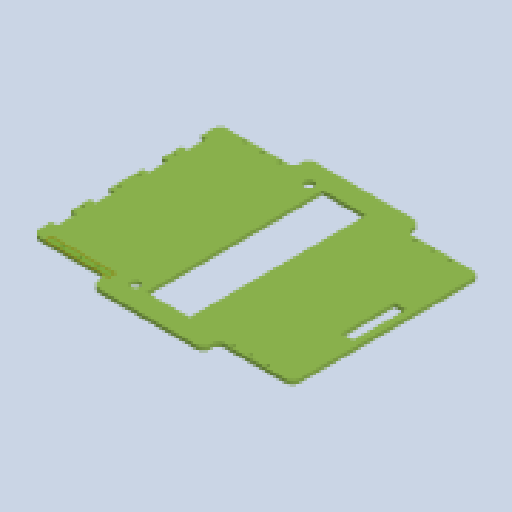
# Autodesk Inventor part: верхняя пластина
Saved by Autodesk Inventor 2024.2 (Build 282272000, 272)
## iProperties
Created: 2025-11-23
Part Number: верхняя пластина
Material: Типовые
Document SubType Name: Modeling
Designer: katya_notebook
Density: 1 g/cm^3
Appearance: Оливково-зеленый
Mass: 177.745 g
Surface Area: 959.322 cm^2
Volume: 177.745 cm^3
Author: katya_notebook
Autodesk Inventor part; units mm, degrees
ref_plane "YZ Plane" through (0, 0, 0) normal (1, 0, 0) x (0, 1, 0)
ref_plane "XZ Plane" through (0, 0, 0) normal (0, 1, 0) x (-1, 0, 0)
ref_plane "XY Plane" through (0, 0, 0) normal (0, 0, 1) x (1, 0, 0)
ref_plane "РабПлоскость1" through (-487.5503, -280.3956, -187.6025) normal (0, -1, 0) x (1, 0, 0)
sketch "Эскиз1" plane through (-487.5503, -280.3956, -187.6025) normal (0, -1, 0) x (1, 0, 0)
  line L0 (-76.4763, 6.5) -> (193.5237, 6.5)
  line L1 (193.5237, 6.5) -> (193.5237, -188.5)
  line L2 (193.5237, -188.5) -> (-76.4763, -188.5)
  line L3 (-76.4763, -188.5) -> (-76.4763, 6.5)
  line L4 (-76.4763, -13.5) -> (-76.4763, -1.5) projected
  circle A0 centre (-12, 3.25) radius 1.75
  circle A1 centre (-48, 3.25) radius 1.75
  circle A2 centre (-30, 3.25) radius 1.75
  line L5 (-76.4763, -91) -> (193.5237, -91)
  circle A3 centre (-12, -185.25) radius 1.75
  circle A4 centre (-48, -185.25) radius 1.75
  circle A5 centre (-30, -185.25) radius 1.75
  point P0 (487.5503, 187.6025)
  point P1 (-60, 3.25)
  dimension "d0" = 195
  dimension "d1" = 270
  dimension "d2" = 0
  dimension "d5" = 3.5
  dimension "d6" = 3.5
  dimension "d8" = 12
  dimension "d9" = 3.25
  dimension "d10" = 3.25
  dimension "d11" = 3.5
  dimension "d12" = 3.25
  dimension "d13" = 18
  dimension "d14" = 97.5
  constraints: 10 end point, 6 centre point, 3 symmetric about line, 2 parallel, 2 perpendicular, 1 horizontal, 1 midpoint, 1 point on line, 3 other
  measures "d0" distance of L0.end L1.end
  measures "d1" distance of L1.end L2.end
  measures "d2" distance between parallel lines of L4 L3
  measures "d5" diameter of A1
  measures "d6" diameter of A0
  measures "d8" distance of A1.centre point (-60, 3.25)
  measures "d9" distance from line of L0 A0.centre
  measures "d10" distance from line of L0 A1.centre
  measures "d11" diameter of A2
  measures "d12" distance from line of L0 A2.centre
  measures "d13" distance of A1.centre A2.centre
  measures "d14" distance between parallel lines of L5 L0
extrude "Выдавливание1" add sketch "Эскиз1" along normal blind 4 contours L0 L1 L5 L3 | L1 L2 L3 L5 | A0 | A1 | A2 | A3 | A4 | A5
sketch "Эскиз2" plane through (-487.5503, -284.3956, -187.6025) normal (0, -1, 0) x (1, 0, 0)
  circle A0 centre (-48, -185.25) radius 1.75 projected
  circle A1 centre (-30, -185.25) radius 1.75 projected
  circle A2 centre (-12, -185.25) radius 1.75 projected
  line L0 (0, -182) -> (-60, -182) projected
  line L1 (-60, -182) -> (-60, -188.5) projected
  line L2 (0, -188.5) -> (-60, -188.5) projected
  line L3 (0, -182) -> (0, -188.5) projected
  circle A3 centre (-48, 3.25) radius 1.75 projected
  circle A4 centre (-30, 3.25) radius 1.75 projected
  circle A5 centre (-12, 3.25) radius 1.75 projected
  line L4 (0, 0) -> (-60, 0) projected
  line L5 (0, 0) -> (0, 6.5) projected
  line L6 (0, 6.5) -> (-60, 6.5) projected
  line L7 (-60, 0) -> (-60, 6.5) projected
  circle A6 centre (165.0475, 3.25) radius 1.75 projected
  circle A7 centre (129.0475, 3.25) radius 1.75 projected
  circle A8 centre (147.0475, 3.25) radius 1.75 projected
  line L8 (116.803, 6.5) -> (116.803, 0) projected
  line L9 (116.803, 0) -> (176.803, 0) projected
  line L10 (176.803, 0) -> (176.803, 6.5) projected
  line L11 (176.803, 6.5) -> (116.803, 6.5) projected
  circle A9 centre (165.0475, -185.25) radius 1.75 projected
  circle A10 centre (129.0475, -185.25) radius 1.75 projected
  circle A11 centre (147.0475, -185.25) radius 1.75 projected
  line L12 (116.803, -188.5) -> (116.803, -182) projected
  line L13 (176.803, -188.5) -> (116.803, -188.5) projected
  line L14 (176.803, -182) -> (176.803, -188.5) projected
  line L15 (116.803, -182) -> (176.803, -182) projected
  line L16 (81.0237, 0.5) -> (81.0237, -182.5) projected
  line L17 (36.0237, 0.5) -> (81.0237, 0.5) projected
  line L18 (36.0237, -182.5) -> (36.0237, 0.5) projected
  line L19 (36.0237, -182.5) -> (81.0237, -182.5) projected
  point P0 (487.5503, 187.6025)
extrude "Выдавливание2" cut sketch "Эскиз2" against normal blind 10 contours A0 | A1 | A2 | A3 | A4 | A5 | A6 | A7 | A8 | A9 | A10 | A11
sketch "Эскиз3" plane through (-487.5503, -284.3956, -187.6025) normal (0, -1, 0) x (1, 0, 0)
  circle A0 centre (23.5237, -1) radius 5 projected
  circle A1 centre (23.5237, -181) radius 5 projected
  line L0 (36.0237, -182.5) -> (36.0237, 0.5) projected
  line L1 (81.0237, 0.5) -> (81.0237, -182.5) projected
  line L2 (36.0237, 0.5) -> (81.0237, 0.5) projected
  line L3 (81.0237, -182.5) -> (36.0237, -182.5) projected
  point P0 (487.5503, 187.6025)
extrude "Выдавливание3" cut sketch "Эскиз3" against normal blind 10
sketch "Эскиз4" plane through (-487.5503, -284.3956, -187.6025) normal (0, -1, 0) x (1, 0, 0)
  arc A0 (116.803, 10.7701) -> (120.803, 6.5) centre (124.2371, 13.7254) ccw projected
  line L0 (116.803, 10.7701) -> (0.2701, 10.7701) projected
  arc A1 (-4, 6.5) -> (0.2701, 10.7701) centre (-7.1034, 13.8735) ccw projected
  arc A2 (0, -192.5) -> (-4, -188.5) centre (-7.2915, -195.7915) ccw projected
  line L1 (0, -192.5) -> (116.803, -192.5) projected
  arc A3 (120.803, -188.5) -> (116.803, -192.5) centre (124.0945, -195.7915) ccw projected
  line L2 (120.803, -188.5) -> (-4, -188.5)
  line L3 (-4, 6.5) -> (120.803, 6.5)
  point P0 (487.5503, 187.6025)
  constraints: 4 end point, 1 horizontal, 1 parallel
extrude "Выдавливание4" add sketch "Эскиз4" against normal blind 4
sketch "Эскиз5" plane through (-487.5503, -284.3956, -187.6025) normal (0, -1, 0) x (1, 0, 0)
  line L0 (174.5237, -118.4235) -> (174.5237, -63.4235) projected
  line L1 (186.5237, -118.4235) -> (174.5237, -118.4235) projected
  line L2 (186.5237, -63.4235) -> (186.5237, -118.4235) projected
  line L3 (174.5237, -63.4235) -> (186.5237, -63.4235) projected
  point P0 (487.5503, 187.6025)
extrude "Выдавливание5" cut sketch "Эскиз5" against normal blind 10
ref_plane "РабПлоскость2" through (-558.0266, -285.3956, -376.1025) normal (1, 0, 0) x (0, 1, 0)
sketch "Эскиз7" plane through (-564.0266, -280.3956, -376.1025) normal (-1, 0, 0) x (0, 0, 1)
  line L0 (175, -5) -> (175, 0) projected
  line L1 (155, 0) -> (155, -5) projected
  line L2 (155, -5) -> (175, -5) projected
  line L3 (195, 0) -> (0, 0) projected
  line L4 (115, -5) -> (135, -5) projected
  line L5 (135, -5) -> (135, 0) projected
  line L6 (115, 0) -> (115, -5) projected
  line L7 (80, -5) -> (80, 0) projected
  line L8 (60, -5) -> (80, -5) projected
  line L9 (60, 0) -> (60, -5) projected
  line L10 (40, -5) -> (40, 0) projected
  line L11 (20, -5) -> (40, -5) projected
  line L12 (20, 0) -> (20, -5) projected
  line L13 (90.375, 55.705) -> (90.375, 55.205) projected
  line L14 (90.375, 55.205) -> (88.875, 55.205) projected
  line L15 (85.375, 55.205) -> (83.875, 55.205) projected
  line L16 (83.875, 55.205) -> (83.875, 55.705) projected
  line L17 (80, 59.705) -> (80, 60.705) projected
  line L18 (80, 60.705) -> (60, 60.705) projected
  line L19 (60, 60.705) -> (60, 59.705) projected
  line L20 (51.75, 55.205) -> (51.75, 47.705) projected
  line L21 (53.25, 55.705) -> (53.25, 55.205) projected
  line L22 (53.25, 55.205) -> (51.75, 55.205) projected
  line L23 (51.75, 47.705) -> (48.25, 47.705) projected
  line L24 (48.25, 47.705) -> (48.25, 55.205) projected
  line L25 (48.25, 55.205) -> (46.75, 55.205) projected
  line L26 (46.75, 55.205) -> (46.75, 55.705) projected
  line L27 (40, 59.705) -> (40, 60.705) projected
  line L28 (40, 60.705) -> (20, 60.705) projected
  line L29 (20, 60.705) -> (20, 59.705) projected
  line L30 (0, 59.705) -> (0, 0) projected
  line L31 (20, 0) -> (0, 0) projected
  line L32 (20, 0) -> (20, -5) projected
  line L33 (20, -5) -> (40, -5) projected
  line L34 (40, -5) -> (40, 0) projected
  line L35 (48.25, 0) -> (40, 0) projected
  line L36 (48.25, 0) -> (48.25, 1.5) projected
  line L37 (48.25, 1.5) -> (46.75, 1.5) projected
  line L38 (46.75, 1.5) -> (46.75, 4.5) projected
  line L39 (46.75, 4.5) -> (48.25, 4.5) projected
  line L40 (48.25, 4.5) -> (48.25, 12) projected
  line L41 (48.25, 12) -> (51.75, 12) projected
  line L42 (51.75, 12) -> (51.75, 4.5) projected
  line L43 (51.75, 4.5) -> (53.25, 4.5) projected
  line L44 (53.25, 4.5) -> (53.25, 1.5) projected
  line L45 (53.25, 1.5) -> (51.75, 1.5) projected
  line L46 (51.75, 1.5) -> (51.75, 0) projected
  line L47 (60, 0) -> (51.75, 0) projected
  line L48 (60, 0) -> (60, -5) projected
  line L49 (60, -5) -> (80, -5) projected
  line L50 (80, -5) -> (80, 0) projected
  line L51 (85.375, 0) -> (80, 0) projected
  line L52 (85.375, 0) -> (85.375, 1.5) projected
  line L53 (85.375, 1.5) -> (83.875, 1.5) projected
  line L54 (83.875, 1.5) -> (83.875, 4.5) projected
  line L55 (83.875, 4.5) -> (85.375, 4.5) projected
  line L56 (88.875, 1.5) -> (88.875, 0) projected
  line L57 (88.875, 4.5) -> (90.375, 4.5) projected
  line L58 (90.375, 4.5) -> (90.375, 1.5) projected
  line L59 (90.375, 1.5) -> (88.875, 1.5) projected
  line L60 (106.125, 0) -> (88.875, 0) projected
  line L61 (115, 0) -> (109.625, 0) projected
  line L62 (106.125, 0) -> (106.125, 1.5) projected
  line L63 (106.125, 1.5) -> (104.625, 1.5) projected
  line L64 (104.625, 1.5) -> (104.625, 4.5) projected
  line L65 (104.625, 4.5) -> (106.125, 4.5) projected
  line L66 (109.625, 1.5) -> (109.625, 0) projected
  line L67 (109.625, 4.5) -> (111.125, 4.5) projected
  line L68 (111.125, 4.5) -> (111.125, 1.5) projected
  line L69 (111.125, 1.5) -> (109.625, 1.5) projected
  line L70 (115, 0) -> (115, -5) projected
  line L71 (115, -5) -> (135, -5) projected
  line L72 (135, -5) -> (135, 0) projected
  line L73 (143.25, 0) -> (135, 0) projected
  line L74 (143.25, 0) -> (143.25, 1.5) projected
  line L75 (143.25, 1.5) -> (141.75, 1.5) projected
  line L76 (141.75, 1.5) -> (141.75, 4.5) projected
  line L77 (141.75, 4.5) -> (143.25, 4.5) projected
  line L78 (143.25, 4.5) -> (143.25, 12) projected
  line L79 (143.25, 12) -> (146.75, 12) projected
  line L80 (146.75, 12) -> (146.75, 4.5) projected
  line L81 (146.75, 4.5) -> (148.25, 4.5) projected
  line L82 (148.25, 4.5) -> (148.25, 1.5) projected
  line L83 (148.25, 1.5) -> (146.75, 1.5) projected
  line L84 (146.75, 1.5) -> (146.75, 0) projected
  line L85 (155, 0) -> (146.75, 0) projected
  line L86 (155, 0) -> (155, -5) projected
  line L87 (155, -5) -> (175, -5) projected
  line L88 (175, -5) -> (175, 0) projected
  line L89 (195, 0) -> (175, 0) projected
  line L90 (195, 59.705) -> (195, 0) projected
  line L91 (175, 59.705) -> (175, 60.705) projected
  line L92 (175, 60.705) -> (155, 60.705) projected
  line L93 (155, 60.705) -> (155, 59.705) projected
  line L94 (146.75, 55.205) -> (146.75, 47.705) projected
  line L95 (148.25, 55.705) -> (148.25, 55.205) projected
  line L96 (148.25, 55.205) -> (146.75, 55.205) projected
  line L97 (146.75, 47.705) -> (143.25, 47.705) projected
  line L98 (143.25, 47.705) -> (143.25, 55.205) projected
  line L99 (143.25, 55.205) -> (141.75, 55.205) projected
  line L100 (141.75, 55.205) -> (141.75, 55.705) projected
  line L101 (135, 59.705) -> (135, 60.705) projected
  line L102 (135, 60.705) -> (115, 60.705) projected
  line L103 (115, 60.705) -> (115, 59.705) projected
  line L104 (111.125, 55.705) -> (111.125, 55.205) projected
  line L105 (111.125, 55.205) -> (109.625, 55.205) projected
  line L106 (106.125, 55.205) -> (104.625, 55.205) projected
  line L107 (104.625, 55.205) -> (104.625, 55.705) projected
  line L108 (175, 55.705) -> (187, 55.705) projected
  line L109 (115, 55.705) -> (111.125, 55.705) projected
  line L110 (104.625, 55.705) -> (90.375, 55.705) projected
  line L111 (83.875, 55.705) -> (80, 55.705) projected
  line L112 (80, 55.705) -> (80, 59.705) projected
  line L113 (60, 59.705) -> (60, 55.705) projected
  line L114 (60, 55.705) -> (53.25, 55.705) projected
  line L115 (46.75, 55.705) -> (40, 55.705) projected
  line L116 (40, 55.705) -> (40, 59.705) projected
  line L117 (155, 59.705) -> (155, 55.705) projected
  line L118 (155, 55.705) -> (148.25, 55.705) projected
  line L119 (141.75, 55.705) -> (135, 55.705) projected
  line L120 (135, 55.705) -> (135, 59.705) projected
  line L121 (115, 59.705) -> (115, 55.705) projected
  line L122 (109.625, 55.205) -> (109.625, 47.705) projected
  line L123 (109.625, 47.705) -> (106.125, 47.705) projected
  line L124 (106.125, 47.705) -> (106.125, 55.205) projected
  line L125 (88.875, 55.205) -> (88.875, 47.705) projected
  line L126 (88.875, 47.705) -> (85.375, 47.705) projected
  line L127 (85.375, 47.705) -> (85.375, 53.705) projected
  line L128 (85.375, 6) -> (85.375, 12) projected
  line L129 (85.375, 12) -> (88.875, 12) projected
  line L130 (106.125, 4.5) -> (106.125, 12) projected
  line L131 (106.125, 12) -> (109.625, 12) projected
  line L132 (109.625, 12) -> (109.625, 4.5) projected
  line L133 (85.375, 6) -> (85.375, 6) projected
  line L134 (88.875, 12) -> (88.875, 4.5) projected
  line L135 (85.375, 53.705) -> (85.375, 53.705) projected
  line L136 (0, 59.705) -> (20, 59.705) projected
  line L137 (85.375, 4.5) -> (85.375, 6) projected
  line L138 (175, 59.705) -> (195, 59.705) projected
  line L139 (85.375, 53.705) -> (85.375, 55.205) projected
  point P0 (376.1025, 280.3956)
  point P1 (88.875, 49.205)
  point P2 (85.375, 49.205)
  point P3 (85.375, 9.5)
  point P4 (106.125, 9.5)
  point P5 (109.625, 9.5)
  point P6 (109.625, 6.5)
  point P7 (109.625, 49.205)
  point P8 (106.125, 49.205)
  point P9 (155, 55.705)
  point P10 (175, 55.705)
  point P11 (115, 55.705)
  point P12 (135, 55.705)
  point P13 (60, 55.705)
  point P14 (80, 55.705)
  point P15 (20, 55.705)
  point P16 (40, 55.705)
  point P17 (20, 0)
  point P18 (40, 0)
  point P19 (60, 0)
  point P20 (80, 0)
  point P21 (135, 0)
  point P22 (46.75, 47.1901)
  dimension "d0" = 195
  dimension "d1" = 270
  dimension "d2" = 0
  dimension "d5" = 3.5
  dimension "d6" = 3.5
  dimension "d8" = 12
  dimension "d9" = 3.25
  dimension "d10" = 3.25
  dimension "d11" = 3.5
  dimension "d12" = 3.25
  dimension "d13" = 18
  dimension "d14" = 97.5
extrude "Выдавливание7" cut sketch "Эскиз7" against normal up to surface (6 mm away) contours L2 L1 L3 L0 | L5 L4 L6 L3 | L7 L8 L9 L3 | L10 L11 L12 L3
sketch "Эскиз8" plane through (-487.5503, -284.3956, -187.6025) normal (0, -1, 0) x (1, 0, 0)
  line L0 (-70.4763, -45.25) -> (-76.4763, -45.25) projected
  line L1 (-76.4763, -40.25) -> (-70.4763, -40.25) projected
  line L2 (-76.4763, -45.25) -> (-76.4763, -41.75) projected
  line L3 (-76.4763, -45.25) -> (-70.4763, -45.25) projected
  line L4 (-70.4763, -41.75) -> (-70.4763, -45.25) projected
  line L5 (-76.4763, -41.75) -> (-70.4763, -41.75) projected
  line L6 (-76.4763, -103.125) -> (-76.4763, -103.125) projected
  line L7 (-76.4763, -103.125) -> (-70.4763, -103.125) projected
  line L8 (-70.4763, -103.125) -> (-70.4763, -103.125) projected
  line L9 (-76.4763, -140.25) -> (-76.4763, -136.75) projected
  line L10 (-76.4763, -140.25) -> (-70.4763, -140.25) projected
  line L11 (-70.4763, -136.75) -> (-70.4763, -140.25) projected
  line L12 (-76.4763, -136.75) -> (-70.4763, -136.75) projected
  circle A0 centre (-73.4763, -43.5) radius 1.75
  circle A1 centre (-73.4763, -80.625) radius 1.75
  circle A2 centre (-73.4763, -101.375) radius 1.75
  circle A3 centre (-73.4763, -138.5) radius 1.75
  line L13 (-76.4763, -103.125) -> (-70.4763, -103.125) projected
  point P0 (487.5503, 187.6025)
  constraints: 4 centre point
extrude "Выдавливание8" cut sketch "Эскиз8" against normal blind 10 contours A0 | A3 | A1 | A2
sketch "Эскиз9" plane through (-487.5503, -284.3956, -187.6025) normal (0, -1, 0) x (1, 0, 0)
  line L0 (0, -192.5) -> (116.803, -192.5) projected
  line L1 (0, -192.5) -> (0, -204)
  line L2 (0, -204) -> (116.803, -204)
  line L3 (116.803, -204) -> (116.803, -192.5)
  line L4 (0, -192.5) -> (116.803, -192.5)
  line L5 (116.803, 10.7701) -> (0.2701, 10.7701) projected
  line L6 (0.2701, 10.7701) -> (116.803, 10.7701)
  line L7 (116.803, 10.7701) -> (116.803, 22.2701)
  line L8 (116.803, 22.2701) -> (0.2701, 22.2701)
  line L9 (0.2701, 22.2701) -> (0.2701, 10.7701)
  point P0 (487.5503, 187.6025)
  point P1 (116.803, 10.7701)
  dimension "d29" = 11.5
  dimension "d30" = 11.5
  constraints: 16 end point, 3 perpendicular, 2 horizontal, 2 parallel, 1 vertical
  measures "d29" distance of L1.end L0.start
  measures "d30" distance of L6.end L7.end
extrude "Выдавливание9" add sketch "Эскиз9" against normal blind 4
fillet "Сопряжение1" radius 8 7 edges at (-487.2802, -282.3956, -165.3324) (-370.7474, -282.3956, -165.3324) (-294.0266, -282.3956, -181.1025) (-294.0266, -282.3956, -376.1025) (-370.7474, -282.3956, -391.6025) (-487.5503, -282.3956, -391.6025) (-564.0266, -282.3956, -376.1025)
fillet "Сопряжение2" radius 8 1 edges at (-564.0266, -282.3956, -181.1025)
